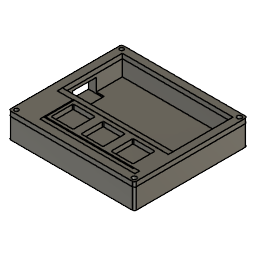
HackPad base stl_ (Autodesk Fusion 360 design; units mm, degrees)
part number: 2026-07-17-21-34-09-282
Autodesk Fusion 360 part; units mm, degrees
sketch "Skizze1" plane through (0, 0, 0) normal (0, 0, 1) x (1, 0, 0)
  line L0 (-25, -35) -> (55, -35)
  line L1 (55, -35) -> (55, 37)
  line L2 (55, 37) -> (-25, 37)
  line L3 (-25, 37) -> (-25, -35)
  line L4 (-20, -30) -> (50.4, -30)
  line L5 (50.4, -30) -> (50.4, 32.4)
  line L6 (50.4, 32.4) -> (-20, 32.4)
  line L7 (-20, 32.4) -> (-20, -30)
  circle A0 centre (52.5, 34.5) radius 1.45
  circle A1 centre (52.5, -32.5) radius 1.45
  circle A2 centre (-22.5, -32.5) radius 1.25
  circle A3 centre (-22.5, 34.5) radius 1.25
  dimension "d1" = 80
  dimension "d2" = 72
  dimension "d3" = 70.4
  dimension "d4" = 62.4
  dimension "d5" = 2.9
  dimension "d6" = 2.5
  dimension "d7" = 2.5
  dimension "d8" = 2.9
  dimension "d9" = 2.5
  dimension "d10" = 2.5
  dimension "d11" = 2.5
  dimension "d12" = 2.5
  dimension "d13" = 2.5
  dimension "d14" = 2.5
  constraint horizontal L0
  constraint vertical L1
  constraint horizontal L2
  constraint vertical L3
  constraint horizontal L4
  constraint vertical L5
  constraint horizontal L6
  constraint vertical L7
  measures "d1" distance of L0.start L0.end
  measures "d2" distance of L0.start L2.end
  measures "d3" distance of L4.start L4.end
  measures "d4" distance of L4.start L6.end
  measures "d5" diameter of A0
  measures "d6" distance of L2 A0.centre
  measures "d7" distance of L1 A0.centre
  measures "d8" diameter of A1
  measures "d9" distance of L1 A1.centre
  measures "d10" distance of L0 A1.centre
  measures "d11" diameter of A2
  measures "d12" diameter of A3
  measures "d13" distance of L2 A3.centre
  measures "d14" distance of L3 A3.centre
extrude "Extrusion1" add sketch "Skizze1" along normal blind 13 makes body 1
extrude "Extrusion2" add sketch "Skizze1" along normal blind 3 contours L4 L5 L6 L7 bodies 1
sketch "Skizze3" plane through (0, 0, 3) normal (0, 0, 1) x (-1, 0, 0)
  line L0 (20, -32.4) -> (20, 30)
  line L1 (20, 30) -> (-50.4, 30)
  line L2 (-50.4, 30) -> (-50.4, -32.4)
  line L3 (-50.4, -32.4) -> (20, -32.4)
sketch "Skizze5" plane through (0, 0, 13) normal (0, 0, 1) x (-1, 0, 0)
  circle A0 centre (22.5, -34.5) radius 1.25
  circle A1 centre (-52.5, -34.5) radius 1.45
  circle A2 centre (22.5, 32.5) radius 1.25
  circle A3 centre (-52.5, 32.5) radius 1.45
  line L0 (20, 30) -> (20, -32.4)
  line L1 (20, -32.4) -> (-50.4, -32.4)
  line L2 (-50.4, -32.4) -> (-50.4, 30)
  line L3 (-50.4, 30) -> (20, 30)
  line L4 (25, -37) -> (25, 35)
  line L5 (25, 35) -> (-55, 35)
  line L6 (-55, 35) -> (-55, -37)
  line L7 (-55, -37) -> (25, -37)
extrude "Extrusion3" add sketch "Skizze5" along normal blind 3 bodies 1
ref_plane "Arbeitsebene1" through (15, 1, 13) normal (0, 0, 1) x (-1, 0, 0)
split "Teilen1" by plane through (15, 1, 13) normal (0, 0, 1) bodies 1 makes body 2 at (3.2775, -32.048, 16)
fillet "Abrundung1" radius 1.2 8 edges at (55, -35, 6.5) (55, 37, 6.5) (-25, 37, 6.5) (-25, -35, 6.5) (55, -35, 14.5) (55, 37, 14.5) (-25, 37, 14.5) (-25, -35, 14.5) on bodies 1 2
move_body "Verschieben1" bodies 2 to x (1, 0, 0) y (0, 1, 0) z (0, 0, 1) at (0, 85, 32)
sketch "Skizze6" plane through (0, 0, 13) normal (0, 0, 1) x (1, 0, 0)
  line L0 (-7.215, -11.175) -> (5.785, -11.175)
  line L1 (-7.215, -25.175) -> (5.785, -25.175)
  line L2 (-7.715, -11.675) -> (-7.715, -24.675)
  line L3 (6.285, -11.675) -> (6.285, -24.675)
  arc A0 (-7.215, -11.175) -> (-7.715, -11.675) centre (-7.215, -11.675) ccw
  arc A1 (6.285, -11.675) -> (5.785, -11.175) centre (5.785, -11.675) ccw
  arc A2 (-7.715, -24.675) -> (-7.215, -25.175) centre (-7.215, -24.675) ccw
  arc A3 (5.785, -25.175) -> (6.285, -24.675) centre (5.785, -24.675) ccw
  line L4 (11.835, -11.175) -> (24.835, -11.175)
  line L5 (11.835, -25.175) -> (24.835, -25.175)
  line L6 (11.335, -11.675) -> (11.335, -24.675)
  line L7 (25.335, -11.675) -> (25.335, -24.675)
  arc A4 (11.835, -11.175) -> (11.335, -11.675) centre (11.835, -11.675) ccw
  arc A5 (25.335, -11.675) -> (24.835, -11.175) centre (24.835, -11.675) ccw
  arc A6 (11.335, -24.675) -> (11.835, -25.175) centre (11.835, -24.675) ccw
  arc A7 (24.835, -25.175) -> (25.335, -24.675) centre (24.835, -24.675) ccw
  line L8 (30.885, -11.175) -> (43.885, -11.175)
  line L9 (30.885, -25.175) -> (43.885, -25.175)
  line L10 (30.385, -11.675) -> (30.385, -24.675)
  line L11 (44.385, -11.675) -> (44.385, -24.675)
  arc A8 (30.885, -11.175) -> (30.385, -11.675) centre (30.885, -11.675) ccw
  arc A9 (44.385, -11.675) -> (43.885, -11.175) centre (43.885, -11.675) ccw
  arc A10 (30.385, -24.675) -> (30.885, -25.175) centre (30.885, -24.675) ccw
  arc A11 (43.885, -25.175) -> (44.385, -24.675) centre (43.885, -24.675) ccw
  line L12 (-10.24, -27.7) -> (46.91, -27.7)
  line L13 (-10.24, -8.65) -> (46.91, -8.65)
  line L14 (-10.24, -27.7) -> (-10.24, -8.65)
  line L15 (46.91, -27.7) -> (46.91, -8.65)
move_body "Verschieben2" bodies 2 to x (1, 0, 0) y (0, 1, 0) z (0, 0, 1) at (0, -85, -32)
extrude "Extrusion4" add sketch "Skizze6" along normal blind 3 separate body makes body 3
move_body "Verschieben3" bodies 3 2 to x (1, 0, 0) y (0, 1, 0) z (0, 0, 1) at (0, 0, 14)
sketch "Skizze7" plane through (0, 0, 13) normal (0, 0, 1) x (-1, 0, 0)
  arc A0 (25, 33.8) -> (23.8, 35) centre (23.8, 33.8) ccw
  line L0 (23.8, 35) -> (-53.8, 35)
  arc A1 (-53.8, 35) -> (-55, 33.8) centre (-53.8, 33.8) ccw
  line L1 (-55, 33.8) -> (-55, -35.8)
  arc A2 (-55, -35.8) -> (-53.8, -37) centre (-53.8, -35.8) ccw
  line L2 (-53.8, -37) -> (23.8, -37)
  arc A3 (23.8, -37) -> (25, -35.8) centre (23.8, -35.8) ccw
  line L3 (25, -35.8) -> (25, 33.8)
  line L4 (-50.4, -32.4) -> (-50.4, 30)
  line L5 (-50.4, 30) -> (20, 30)
  line L6 (20, 30) -> (20, -32.4)
  line L7 (20, -32.4) -> (-50.4, -32.4)
  circle A4 centre (-52.5, 32.5) radius 1.45
  circle A5 centre (22.5, 32.5) radius 1.25
  circle A6 centre (-52.5, -34.5) radius 1.45
  circle A7 centre (22.5, -34.5) radius 1.25
  line L8 (10, 9) -> (21, 9)
  line L9 (21, 9) -> (21, 30)
  line L10 (21, 30) -> (10, 30)
  line L11 (10, 30) -> (10, 9)
  line L12 (10, 30) -> (-50.4, 30)
  line L13 (-50.4, 30) -> (-50.4, 27.0742)
  line L14 (-50.4, 27.0742) -> (10, 27.0742)
  line L15 (10, 27.0742) -> (10, 30)
  line L16 (-50.4, 27.0742) -> (-46.389, 27.0742)
  line L17 (-46.389, 27.0742) -> (-46.389, 8.7494)
  line L18 (-46.389, 8.7494) -> (-50.4, 8.7494)
  line L19 (-50.4, 8.7494) -> (-50.4, 27.0742)
  line L20 (-50.4, 8.7494) -> (23.716, 8.7494)
  line L21 (23.716, 8.7494) -> (23.716, 5.7494)
  line L22 (23.716, 5.7494) -> (-50.4, 5.7494)
  line L23 (-50.4, 5.7494) -> (-50.4, 8.7494)
  line L24 (9.4695, 8.2191) -> (21.7625, 8.2191)
  line L25 (21.7625, 8.2191) -> (21.7625, 30.4276)
  line L26 (21.7625, 30.4276) -> (9.4695, 30.4276)
  line L27 (9.4695, 30.4276) -> (9.4695, 8.2191)
  dimension "d29" = 3
  constraint horizontal L8
  constraint vertical L9
  constraint horizontal L10
  constraint vertical L11
  constraint horizontal L12
  constraint vertical L13
  constraint horizontal L14
  constraint vertical L15
  constraint coincident L4 L13.end
  constraint horizontal L16
  constraint vertical L17
  constraint horizontal L18
  constraint vertical L19
  constraint horizontal L20
  constraint vertical L21
  constraint horizontal L22
  constraint vertical L23
  constraint horizontal L24
  constraint vertical L25
  constraint horizontal L26
  constraint vertical L27
  measures "d29" distance of L18.end L22.end
extrude "Extrusion5" add sketch "Skizze7" along normal blind 3 separate body contours L6 L8 L11 L14 L20 L27 makes body 4
extrude "Extrusion6" add sketch "Skizze7" along normal blind 3 separate body contours L4 L6 L18 L20 L22 L23 L24 L27 makes body 5
extrude "Extrusion7" add sketch "Skizze7" along normal blind 3 contours L6 L20 L24 L27 bodies 1 4 5
extrude "Extrusion8" add sketch "Skizze7" along normal blind 3 separate body contours L5 L11 L12 L14 L15 L27 makes body 6
extrude "Extrusion9" add sketch "Skizze7" along normal blind 3 contours L4 L5 L12 L13 L14 L16 L27 bodies 1 6
extrude "Extrusion10" add sketch "Skizze7" along normal blind 3 separate body contours L5 L6 L8 L10 L11 L15 makes body 7
extrude "Extrusion11" add sketch "Skizze7" along normal blind 3 separate body contours L4 L14 L16 L17 L18 L19 L20 makes body 8
move_body "Verschieben4" bodies 2 3 to x (1, 0, 0) y (0, 1, 0) z (0, 0, 1) at (0, 0, -14)
sketch "Skizze8" plane through (-25, 0, 0) normal (-1, 0, 0) x (0, -1, 0)
  line L0 (33.8, 0) -> (33.8, 13)
  line L1 (33.8, 13) -> (-35.8, 13)
  line L2 (-35.8, 13) -> (-35.8, 0)
  line L3 (-35.8, 0) -> (33.8, 0)
  line L4 (-15.8, 2.0558) -> (-0.8, 2.0558)
  line L5 (-0.8, 2.0558) -> (-0.8, 11)
  line L6 (-0.8, 11) -> (-15.8, 11)
  line L7 (-15.8, 11) -> (-15.8, 2.0558)
  dimension "d45" = 15
  constraint horizontal L4
  constraint vertical L5
  constraint horizontal L6
  constraint vertical L7
  measures "d45" distance of L4.start L4.end
extrude "Extrusion12" cut sketch "Skizze8" against normal blind 10 contours L4 L5 L6 L7 bodies 1
combine "Kombinieren1" operation add target body 2 tool bodies 3 7
combine "Kombinieren2" operation add target body 2 tool bodies 8
